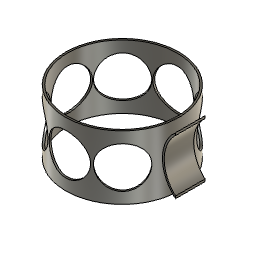
bottle-holder v3 (Autodesk Fusion 360 design; units mm, degrees)
Autodesk Fusion 360 part; units mm, degrees
note: some values were not read from the file. Set by a fixed rule: which sketch regions a step uses.
sketch "Sketch1" plane through (0, 0, 0) normal (0, 0, 1) x (1, 0, 0) in component "maincomp"
  circle A0 centre (0, 0) radius 46.5
  circle A1 centre (0, 0) radius 48
  dimension "d1" = 93
  dimension "d2" = 96
  constraint coincident A0.centre A1.centre
  constraint concentric A0 A1
  measures "d1" diameter of A0
  measures "d2" diameter of A1
extrude "Extrude1" add sketch "Sketch1" along normal blind 65 makes body 1 in component "maincomp"
sketch "Sketch2" plane through (0, 0, 0) normal (1, 0, 0) x (0, 1, 0) in component "maincomp"
ref_plane "WorkPlane1" through (47, 0, 0) normal (1, 0, 0) x (0, 1, 0) in component "maincomp"
sketch "Sketch3" plane through (0, 0, 0) normal (0, 1, 0) x (1, 0, 0) in component "maincomp"
  line L0 (0, 0) -> (78.5, 0)
  line L1 (78.5, 0) -> (78.5, -35)
  line L2 (78.5, -35) -> (0, -35)
  line L3 (0, -35) -> (0, 0)
  circle A0 centre (78.5, -35) radius 30.5
  circle A1 centre (78.5, -35) radius 32
  line L4 (57.5876, -74.0763) -> (121.2006, -74.0763)
  line L5 (121.2006, -74.0763) -> (121.2006, 7.9237)
  line L6 (121.2006, 7.9237) -> (57.5876, 7.9237)
  line L7 (57.5876, 7.9237) -> (57.5876, -74.0763)
  dimension "d6" = 78.5
  dimension "d7" = 35
  dimension "d8" = 61
  dimension "d10" = 64
  dimension "d11" = 63.613
  dimension "d12" = 82
  constraint horizontal L0
  constraint vertical L1
  constraint horizontal L2
  constraint vertical L3
  constraint coincident L0.start L3.end
  constraint coincident L1.end L2.start
  constraint concentric A0 A1
  constraint horizontal L4
  constraint vertical L5
  constraint horizontal L6
  constraint vertical L7
  measures "d6" distance of L0.start L0.end
  measures "d7" distance of L0.start L2.end
  measures "d8" diameter of A0
  measures "d10" diameter of A1
  measures "d11" distance of L4.start L4.end
  measures "d12" distance of L4.start L6.end
extrude "Extrude2" add sketch "Sketch3" along normal mid plane 25 contours L2 A0 A1 L7 | L2 A0 A1 L7 bodies 1 in component "maincomp"
sketch "Sketch4" plane through (0, 0, 0) normal (0, 1, 0) x (1, 0, 0) in component "maincomp"
  circle A0 centre (0.1757, -32.4995) radius 17.5
  dimension "d15" = 35
  dimension "d16" = 32.5
  measures "d15" diameter of A0
  measures "d16" distance of origin A0.centre
extrude "Extrude3" add sketch "Sketch4" along normal mid plane 200 separate body makes body 2 in component "maincomp"
copy_body "CopyPasteBodies3" bodies 2 makes body 3 in component "maincomp"
move_body "Move3" bodies 3 to x (0, 1, 0) y (-1, 0, 0) z (0, 0, 1) at (0, 0, 0) in component "maincomp"
move_body "Move4" bodies 3 to x (1, 0, 0) y (0, 1, 0) z (0, 0, 1) at (-100, 0, 0) in component "maincomp"
copy_body "CopyPasteBodies1" bodies 2 makes body 4 in component "maincomp"
move_body "Move1" bodies 4 to x (0.707107, 0.707107, 0) y (-0.707107, 0.707107, 0) z (0, 0, 1) at (0, 0, 0) in component "maincomp"
copy_body "CopyPasteBodies2" bodies 2 makes body 5 in component "maincomp"
move_body "Move2" bodies 5 to x (0.707107, -0.707107, 0) y (0.707107, 0.707107, 0) z (0, 0, 1) at (0, 0, 0) in component "maincomp"
combine "Combine1" operation cut target body 1 tool bodies 2 3 4 5 in component "maincomp"
ref_plane "WorkPlane2" through (0, 0, 32.5) normal (0, 0, 1) x (1, 0, 0) in component "maincomp"
sketch "Sketch5" plane through (0, 0, 32.5) normal (0, 0, 1) x (1, 0, 0) in component "maincomp"
  circle A0 centre (0, 0) radius 75
  dimension "d24" = 150
  constraint coincident A0.centre origin
  measures "d24" diameter of A0
extrude "Extrude4" add sketch "Sketch5" along normal mid plane 54 separate body makes body 6 in component "maincomp"
combine "Combine2" operation intersect target body 1 tool bodies 6 in component "maincomp"
component "maincomp" placed x (1, 0, 0) y (0, 1, 0) z (0, 0, 1) at (0, 0, 0)
equation "d6 = 48 mm + bottleid / 2"
equation "d8 = bottleid"
equation "bottleid = 61 mm"
equation "d10 = bottleid + 3 mm"
